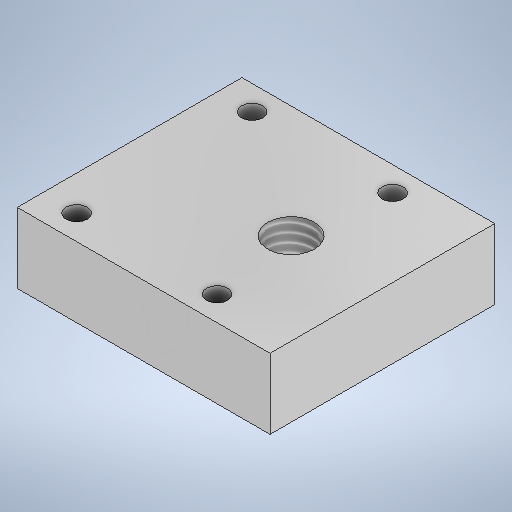
# Autodesk Inventor part: LM Cart Braket
Saved by Autodesk Inventor 2026.2 (Build 302298010, 298A)
## iProperties
Created: 2026-04-29
Part Number: LM Cart Braket
Material: Aluminum 6061-AHC
Document SubType Name: Modeling
Designer: chanh
Density: 2.7 g/cm^3
Appearance: Aluminum - Dark
Author: chanh
Autodesk Inventor part; units mm, degrees
ref_plane "YZ Plane" through (0, 0, 0) normal (1, 0, 0) x (0, 1, 0)
ref_plane "XZ Plane" through (0, 0, 0) normal (0, 1, 0) x (-1, 0, 0)
ref_plane "XY Plane" through (0, 0, 0) normal (0, 0, 1) x (1, 0, 0)
sketch "Sketch1" plane through (0, 0, 0) normal (0, 1, 0) x (-1, 0, 0)
  line L0 (18, 16) -> (-18, 16)
  line L1 (-18, 16) -> (-18, -16)
  line L2 (-18, -16) -> (18, -16)
  line L3 (18, -16) -> (18, 16)
  line L4 (18, 16) -> (-18, -16) construction
  line L5 (-18, 16) -> (18, -16) construction
  point P0 (0, 0)
  dimension "d0" = 36
  dimension "d1" = 32
  constraints: 12 end point, 2 midpoint, 2 parallel, 1 horizontal, 1 perpendicular
  measures "d0" distance of L2.end L1.end
  measures "d1" distance of L1.end L0.end
extrude "Extrusion1" add sketch "Sketch1" along normal blind 10
sketch "Sketch2" plane through (0, 0, 0) normal (0, -1, 0) x (1, 0, 0)
  circle A0 centre (6.95, 12.5) radius 1.2295 projected
  circle A1 centre (6.95, -12.5) radius 1.2295 projected
  circle A2 centre (-13.05, -12.5) radius 1.2295 projected
  circle A3 centre (-13.05, 12.5) radius 1.2295 projected
  line L0 (-24.1, 15) -> (18, 15) projected
  line L1 (-24.1, -15) -> (-24.1, 15) projected
  line L2 (18, -15) -> (-24.1, -15) projected
  line L3 (18, 15) -> (18, -15) projected
  point P0 (0, 0)
hole "Hole1" at (6.95, 0, -12.5) at (-13.05, 0, -12.5) at (6.95, 0, 12.5) at (-13.05, 0, 12.5) direction (0, 1, 0) diameter 3 end through all counterbore diameter 6 counterbore depth 3.5
sketch "Sketch3" plane through (0, 0, 0) normal (0, -1, 0) x (1, 0, 0)
  circle A0 centre (-13.05, 12.5) radius 3 projected
  circle A1 centre (6.95, 12.5) radius 3 projected
  circle A2 centre (-13.05, -12.5) radius 3 projected
  circle A3 centre (6.95, -12.5) radius 3 projected
  line L0 (18, 16) -> (18, -16) projected
  line L1 (-18, 16) -> (18, 16) projected
  line L2 (-18, -16) -> (-18, 16) projected
  line L3 (18, -16) -> (-18, -16) projected
  point P0 (0, 0)
  point P1 (5, 0)
  dimension "d11" = 5
  constraints: 1 horizontal alignment
  measures "d11" distance of point (0, 0) point (5, 0)
hole "Hole2" at (5, 0, 0) direction (0, 1, 0) diameter 6.647 end through all thread size "M8x1.25" class "6H" standard "ISO Metric profile"
body "Solid1"
